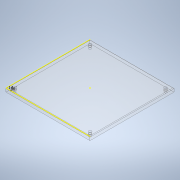
# Autodesk Inventor part: Arrow Panel
Saved by Autodesk Inventor 2021 (Build 250183000, 183)
## iProperties
Created: 2020-11-09
Part Number: Arrow Panel
Material: Polycarbonate, Clear
Document SubType Name: Modeling
Designer: Wes
Density: 1.2 g/cm^3
Appearance: Polycarbonate - Clear
Mass: 1081.09 g
Surface Area: 1633.04 cm^2
Volume: 900.912 cm^3
Author: Wes
Autodesk Inventor part; units mm, degrees
ref_plane "YZ Plane" through (0, 0, 0) normal (1, 0, 0) x (0, 1, 0)
ref_plane "XZ Plane" through (0, 0, 0) normal (0, 1, 0) x (-1, 0, 0)
ref_plane "XY Plane" through (0, 0, 0) normal (0, 0, 1) x (1, 0, 0)
sketch "Sketch1" plane through (0, 0, 0) normal (0, 1, 0) x (-1, 0, 0)
  line L0 (-138, 138) -> (138, 138)
  line L1 (138, 138) -> (138, -138)
  line L2 (138, -138) -> (-138, -138)
  line L3 (-138, -138) -> (-138, 138)
  line L4 (-138, 138) -> (138, -138) construction
  line L5 (138, 138) -> (-138, -138) construction
  line L6 (138, 130.5) -> (130.5, 130.5)
  line L7 (130.5, 130.5) -> (130.5, 138)
  point P0 (0, 0)
  dimension "d0" = 276
  dimension "d1" = 276
  dimension "d18" = 7.5
  constraints: 16 end point, 3 perpendicular, 2 horizontal, 2 midpoint, 2 parallel, 2 point on line
  measures "d0" distance of L1.end L2.end
  measures "d1" distance of L0.end L1.end
  measures "d18" distance of L6.start L6.end
extrude "Extrusion1" add sketch "Sketch1" along normal blind 12
sketch "Sketch3" plane through (0, 12, 0) normal (0, 1, 0) x (1, 0, 0)
  line L0 (-138, 138) -> (-138, -138) projected
  line L1 (-138, -138) -> (138, -138) projected
  point P0 (0, 0)
  point P1 (-124, -124)
  dimension "d21" = 14
  dimension "d22" = 14
  measures "d21" distance from line of L0 point (-124, -124)
  measures "d22" distance from line of L1 point (-124, -124)
hole "Hole2" at (-124, 12, 124) direction (0, -1, 0) diameter 7.94 end through all counterbore diameter 9.53 counterbore depth 6
mirror "Mirror1 Right" about plane through (0, 0, 0) normal (0, 0, 1) of "Hole2"
mirror "Mirror2 Bottom" about plane through (0, 0, 0) normal (1, 0, 0) of "Hole2", "Mirror1 Right"
fillet "Fillet1" radius 2 4 edges at (0, 12, 138) (-138, 12, 0) (138, 12, 0) (0, 12, -138)
body "Solid1"
